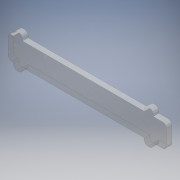
# Autodesk Inventor part: BBGW Case Side
Saved by Autodesk Inventor 2016 (Build 200138000, 138)
## iProperties
Created: 2016-06-26
Part Number: BBGW Case Side
Material: Acrylic, Clear
Document SubType Name: Modeling
Designer: Jacob
Density: 1.19 g/cm^3
Appearance: Transparent - Clear
Author: Jacob
Autodesk Inventor part; units mm, degrees
(part 1 of 2)
ref_plane "YZ Plane" through (0, 0, 0) normal (1, 0, 0) x (0, 1, 0)
ref_plane "XZ Plane" through (0, 0, 0) normal (0, 1, 0) x (-1, 0, 0)
ref_plane "XY Plane" through (0, 0, 0) normal (0, 0, 1) x (1, 0, 0)
sketch "Sketch1" plane through (0, 0, 0) normal (0, 1, 0) x (-1, 0, 0)
  line L0 (176.9998, 77.9421) -> (176.9999, 86.5421)
  spline S0 degree 3 poles (176.9999, 86.5421) (176.9999, 87.6467) (176.1044, 88.5421) (174.9999, 88.5421) knots 0 0 0 0 1 1 1 1
  line L1 (176.9999, 86.5421) -> (176.9999, 87.6467) construction
  line L2 (176.9999, 87.6467) -> (176.1044, 88.5421) construction
  line L3 (176.1044, 88.5421) -> (174.9999, 88.5421) construction
  line L4 (174.9999, 88.5421) -> (173.9998, 88.5421)
  line L5 (173.9998, 88.5421) -> (173.9998, 90.5421)
  line L6 (173.9998, 90.5421) -> (173.9993, 90.5762)
  line L7 (173.9993, 90.5762) -> (173.9975, 90.6103)
  line L8 (173.9975, 90.6103) -> (173.9946, 90.6444)
  line L9 (173.9946, 90.6444) -> (173.9905, 90.6783)
  line L10 (173.9905, 90.6783) -> (173.9853, 90.712)
  line L11 (173.9853, 90.712) -> (173.9789, 90.7456)
  line L12 (173.9789, 90.7456) -> (173.9714, 90.7789)
  line L13 (173.9714, 90.7789) -> (173.9628, 90.8119)
  line L14 (173.9628, 90.8119) -> (173.953, 90.8446)
  line L15 (173.953, 90.8446) -> (173.9421, 90.877)
  line L16 (173.9421, 90.877) -> (173.9301, 90.909)
  line L17 (173.9301, 90.909) -> (173.9171, 90.9405)
  line L18 (173.9171, 90.9405) -> (173.9029, 90.9716)
  line L19 (173.9029, 90.9716) -> (173.8877, 91.0022)
  line L20 (173.8877, 91.0022) -> (173.8715, 91.0322)
  line L21 (173.8715, 91.0322) -> (173.8543, 91.0617)
  line L22 (173.8543, 91.0617) -> (173.836, 91.0906)
  line L23 (173.836, 91.0906) -> (173.8168, 91.1188)
  line L24 (173.8168, 91.1188) -> (173.7967, 91.1463)
  line L25 (173.7967, 91.1463) -> (173.7756, 91.1732)
  line L26 (173.7756, 91.1732) -> (173.7536, 91.1993)
  line L27 (173.7536, 91.1993) -> (173.7307, 91.2247)
  line L28 (173.7307, 91.2247) -> (173.707, 91.2492)
  line L29 (173.707, 91.2492) -> (173.6824, 91.2729)
  line L30 (173.6824, 91.2729) -> (173.6571, 91.2958)
  line L31 (173.6571, 91.2958) -> (173.6309, 91.3178)
  line L32 (173.6309, 91.3178) -> (173.6041, 91.3389)
  line L33 (173.6041, 91.3389) -> (173.5765, 91.3591)
  line L34 (173.5765, 91.3591) -> (173.5483, 91.3783)
  line L35 (173.5483, 91.3783) -> (173.5194, 91.3965)
  line L36 (173.5194, 91.3965) -> (173.49, 91.4138)
  line L37 (173.49, 91.4138) -> (173.4599, 91.43)
  line L38 (173.4599, 91.43) -> (173.4293, 91.4452)
  line L39 (173.4293, 91.4452) -> (173.3983, 91.4593)
  line L40 (173.3983, 91.4593) -> (173.3667, 91.4724)
  line L41 (173.3667, 91.4724) -> (173.3347, 91.4844)
  line L42 (173.3347, 91.4844) -> (173.3024, 91.4952)
  line L43 (173.3024, 91.4952) -> (173.2696, 91.505)
  line L44 (173.2696, 91.505) -> (173.2366, 91.5137)
  line L45 (173.2366, 91.5137) -> (173.2033, 91.5212)
  line L46 (173.2033, 91.5212) -> (173.1698, 91.5276)
  line L47 (173.1698, 91.5276) -> (173.136, 91.5328)
  line L48 (173.136, 91.5328) -> (173.1021, 91.5369)
  line L49 (173.1021, 91.5369) -> (173.0681, 91.5398)
  line L50 (173.0681, 91.5398) -> (173.034, 91.5415)
  line L51 (173.034, 91.5415) -> (172.9999, 91.5421)
  line L52 (172.9999, 91.5421) -> (169.9998, 91.5421)
  line L53 (169.9998, 91.5421) -> (169.9657, 91.5415)
  line L54 (169.9657, 91.5415) -> (169.9316, 91.5398)
  line L55 (169.9316, 91.5398) -> (169.8976, 91.5369)
  line L56 (169.8976, 91.5369) -> (169.8637, 91.5328)
  line L57 (169.8637, 91.5328) -> (169.8299, 91.5276)
  line L58 (169.8299, 91.5276) -> (169.7964, 91.5212)
  line L59 (169.7964, 91.5212) -> (169.7631, 91.5137)
  line L60 (169.7631, 91.5137) -> (169.7301, 91.505)
  line L61 (169.7301, 91.505) -> (169.6973, 91.4952)
  line L62 (169.6973, 91.4952) -> (169.665, 91.4844)
  line L63 (169.665, 91.4844) -> (169.633, 91.4724)
  line L64 (169.633, 91.4724) -> (169.6014, 91.4593)
  line L65 (169.6014, 91.4593) -> (169.5704, 91.4452)
  line L66 (169.5704, 91.4452) -> (169.5398, 91.43)
  line L67 (169.5398, 91.43) -> (169.5097, 91.4138)
  line L68 (169.5097, 91.4138) -> (169.4803, 91.3965)
  line L69 (169.4803, 91.3965) -> (169.4514, 91.3783)
  line L70 (169.4514, 91.3783) -> (169.4232, 91.3591)
  line L71 (169.4232, 91.3591) -> (169.3956, 91.3389)
  line L72 (169.3956, 91.3389) -> (169.3688, 91.3178)
  line L73 (169.3688, 91.3178) -> (169.3426, 91.2958)
  line L74 (169.3426, 91.2958) -> (169.3173, 91.2729)
  line L75 (169.3173, 91.2729) -> (169.2927, 91.2492)
  line L76 (169.2927, 91.2492) -> (169.269, 91.2247)
  line L77 (169.269, 91.2247) -> (169.2461, 91.1993)
  line L78 (169.2461, 91.1993) -> (169.2241, 91.1732)
  line L79 (169.2241, 91.1732) -> (169.203, 91.1463)
  line L80 (169.203, 91.1463) -> (169.1829, 91.1188)
  line L81 (169.1829, 91.1188) -> (169.1637, 91.0906)
  line L82 (169.1637, 91.0906) -> (169.1454, 91.0617)
  line L83 (169.1454, 91.0617) -> (169.1282, 91.0322)
  line L84 (169.1282, 91.0322) -> (169.112, 91.0022)
  line L85 (169.112, 91.0022) -> (169.0968, 90.9716)
  line L86 (169.0968, 90.9716) -> (169.0826, 90.9405)
  line L87 (169.0826, 90.9405) -> (169.0696, 90.909)
  line L88 (169.0696, 90.909) -> (169.0576, 90.877)
  line L89 (169.0576, 90.877) -> (169.0467, 90.8446)
  line L90 (169.0467, 90.8446) -> (169.0369, 90.8119)
  line L91 (169.0369, 90.8119) -> (169.0283, 90.7789)
  line L92 (169.0283, 90.7789) -> (169.0208, 90.7456)
  line L93 (169.0208, 90.7456) -> (169.0144, 90.712)
  line L94 (169.0144, 90.712) -> (169.0092, 90.6783)
  line L95 (169.0092, 90.6783) -> (169.0051, 90.6444)
  line L96 (169.0051, 90.6444) -> (169.0022, 90.6103)
  line L97 (169.0022, 90.6103) -> (169.0004, 90.5762)
  line L98 (169.0004, 90.5762) -> (168.9998, 90.5421)
  line L99 (168.9998, 90.5421) -> (168.9998, 88.5421)
  line L100 (168.9998, 88.5421) -> (102.1834, 88.5421)
  line L101 (102.1834, 88.5421) -> (102.1834, 90.5421)
  line L102 (102.1834, 90.5421) -> (102.1829, 90.5762)
  line L103 (102.1829, 90.5762) -> (102.1811, 90.6103)
  line L104 (102.1811, 90.6103) -> (102.1782, 90.6444)
  line L105 (102.1782, 90.6444) -> (102.1741, 90.6783)
  line L106 (102.1741, 90.6783) -> (102.1689, 90.712)
  line L107 (102.1689, 90.712) -> (102.1625, 90.7456)
  line L108 (102.1625, 90.7456) -> (102.155, 90.7789)
  line L109 (102.155, 90.7789) -> (102.1464, 90.8119)
  line L110 (102.1464, 90.8119) -> (102.1366, 90.8446)
  line L111 (102.1366, 90.8446) -> (102.1257, 90.877)
  line L112 (102.1257, 90.877) -> (102.1137, 90.909)
  line L113 (102.1137, 90.909) -> (102.1007, 90.9405)
  line L114 (102.1007, 90.9405) -> (102.0865, 90.9716)
  line L115 (102.0865, 90.9716) -> (102.0713, 91.0022)
  line L116 (102.0713, 91.0022) -> (102.0551, 91.0322)
  line L117 (102.0551, 91.0322) -> (102.0379, 91.0617)
  line L118 (102.0379, 91.0617) -> (102.0196, 91.0906)
  line L119 (102.0196, 91.0906) -> (102.0004, 91.1188)
  line L120 (102.0004, 91.1188) -> (101.9802, 91.1463)
  line L121 (101.9802, 91.1463) -> (101.9592, 91.1732)
  line L122 (101.9592, 91.1732) -> (101.9372, 91.1993)
  line L123 (101.9372, 91.1993) -> (101.9143, 91.2247)
  line L124 (101.9143, 91.2247) -> (101.8905, 91.2492)
  line L125 (101.8905, 91.2492) -> (101.866, 91.2729)
  line L126 (101.866, 91.2729) -> (101.8406, 91.2958)
  line L127 (101.8406, 91.2958) -> (101.8145, 91.3178)
  line L128 (101.8145, 91.3178) -> (101.7877, 91.3389)
  line L129 (101.7877, 91.3389) -> (101.7601, 91.3591)
  line L130 (101.7601, 91.3591) -> (101.7319, 91.3783)
  line L131 (101.7319, 91.3783) -> (101.703, 91.3965)
  line L132 (101.703, 91.3965) -> (101.6735, 91.4138)
  line L133 (101.6735, 91.4138) -> (101.6435, 91.43)
  line L134 (101.6435, 91.43) -> (101.6129, 91.4452)
  line L135 (101.6129, 91.4452) -> (101.5818, 91.4593)
  line L136 (101.5818, 91.4593) -> (101.5503, 91.4724)
  line L137 (101.5503, 91.4724) -> (101.5183, 91.4844)
  line L138 (101.5183, 91.4844) -> (101.486, 91.4952)
  line L139 (101.486, 91.4952) -> (101.4532, 91.505)
  line L140 (101.4532, 91.505) -> (101.4202, 91.5137)
  line L141 (101.4202, 91.5137) -> (101.3869, 91.5212)
  line L142 (101.3869, 91.5212) -> (101.3533, 91.5276)
  line L143 (101.3533, 91.5276) -> (101.3196, 91.5328)
  line L144 (101.3196, 91.5328) -> (101.2857, 91.5369)
  line L145 (101.2857, 91.5369) -> (101.2517, 91.5398)
  line L146 (101.2517, 91.5398) -> (101.2176, 91.5415)
  line L147 (101.2176, 91.5415) -> (101.1834, 91.5421)
  line L148 (101.1834, 91.5421) -> (98.1834, 91.5421)
  line L149 (98.1834, 91.5421) -> (98.1493, 91.5415)
  line L150 (98.1493, 91.5415) -> (98.1152, 91.5398)
  line L151 (98.1152, 91.5398) -> (98.0812, 91.5369)
  line L152 (98.0812, 91.5369) -> (98.0473, 91.5328)
  line L153 (98.0473, 91.5328) -> (98.0135, 91.5276)
  line L154 (98.0135, 91.5276) -> (97.98, 91.5212)
  line L155 (97.98, 91.5212) -> (97.9467, 91.5137)
  line L156 (97.9467, 91.5137) -> (97.9136, 91.505)
  line L157 (97.9136, 91.505) -> (97.8809, 91.4952)
  line L158 (97.8809, 91.4952) -> (97.8486, 91.4844)
  line L159 (97.8486, 91.4844) -> (97.8166, 91.4724)
  line L160 (97.8166, 91.4724) -> (97.785, 91.4593)
  line L161 (97.785, 91.4593) -> (97.754, 91.4452)
  line L162 (97.754, 91.4452) -> (97.7234, 91.43)
  line L163 (97.7234, 91.43) -> (97.6933, 91.4138)
  line L164 (97.6933, 91.4138) -> (97.6639, 91.3965)
  line L165 (97.6639, 91.3965) -> (97.635, 91.3783)
  line L166 (97.635, 91.3783) -> (97.6068, 91.3591)
  line L167 (97.6068, 91.3591) -> (97.5792, 91.3389)
  line L168 (97.5792, 91.3389) -> (97.5524, 91.3178)
  line L169 (97.5524, 91.3178) -> (97.5262, 91.2958)
  line L170 (97.5262, 91.2958) -> (97.5009, 91.2729)
  line L171 (97.5009, 91.2729) -> (97.4763, 91.2492)
  line L172 (97.4763, 91.2492) -> (97.4526, 91.2247)
  line L173 (97.4526, 91.2247) -> (97.4297, 91.1993)
  line L174 (97.4297, 91.1993) -> (97.4077, 91.1732)
  line L175 (97.4077, 91.1732) -> (97.3866, 91.1463)
  line L176 (97.3866, 91.1463) -> (97.3665, 91.1188)
  line L177 (97.3665, 91.1188) -> (97.3473, 91.0906)
  line L178 (97.3473, 91.0906) -> (97.329, 91.0617)
  line L179 (97.329, 91.0617) -> (97.3118, 91.0322)
  line L180 (97.3118, 91.0322) -> (97.2956, 91.0022)
  line L181 (97.2956, 91.0022) -> (97.2804, 90.9716)
  line L182 (97.2804, 90.9716) -> (97.2662, 90.9405)
  line L183 (97.2662, 90.9405) -> (97.2532, 90.909)
  line L184 (97.2532, 90.909) -> (97.2412, 90.877)
  line L185 (97.2412, 90.877) -> (97.2303, 90.8446)
  line L186 (97.2303, 90.8446) -> (97.2205, 90.8119)
  line L187 (97.2205, 90.8119) -> (97.2119, 90.7789)
  line L188 (97.2119, 90.7789) -> (97.2044, 90.7456)
  line L189 (97.2044, 90.7456) -> (97.198, 90.712)
  line L190 (97.198, 90.712) -> (97.1928, 90.6783)
  line L191 (97.1928, 90.6783) -> (97.1887, 90.6444)
  line L192 (97.1887, 90.6444) -> (97.1858, 90.6103)
  line L193 (97.1858, 90.6103) -> (97.184, 90.5762)
  line L194 (97.184, 90.5762) -> (97.1834, 90.5421)
  line L195 (97.1834, 90.5421) -> (97.1834, 88.5421)
  line L196 (97.1834, 88.5421) -> (92, 88.5421)
  spline S1 degree 3 poles (92, 88.5421) (91.4695, 88.5421) (90.9608, 88.3314) (90.5857, 87.9563) knots 0 0 0 0 0.5 0.5 0.5 0.5
  line L197 (92, 88.5421) -> (91.4695, 88.5421) construction
  line L198 (91.4695, 88.5421) -> (90.9608, 88.3314) construction
  line L199 (90.9608, 88.3314) -> (90.5857, 87.9563) construction
  spline S2 degree 3 poles (90.5857, 87.9563) (90.585325, 87.955925) (90.2107, 87.5812) (90, 87.0725) (90, 86.5421) knots 0.5 0.5 0.5 0.5 0.50000001 1 1 1 1
  line L200 (90.5857, 87.9563) -> (90.5857, 87.9563) construction
  line L201 (90.5857, 87.9563) -> (90.2107, 87.5812) construction
  line L202 (90.2107, 87.5812) -> (90, 87.0725) construction
  line L203 (90, 87.0725) -> (90, 86.5421) construction
  line L204 (90, 86.5421) -> (89.9999, 77.9421)
  spline S3 degree 3 poles (89.9999, 77.9421) (89.9999, 77.4117) (90.2107, 76.903) (90.5857, 76.5279) knots 0 0 0 0 0.5 0.5 0.5 0.5
  line L205 (89.9999, 77.9421) -> (89.9999, 77.4117) construction
  line L206 (89.9999, 77.4117) -> (90.2107, 76.903) construction
  line L207 (90.2107, 76.903) -> (90.5857, 76.5279) construction
  spline S4 degree 3 poles (90.5857, 76.5279) (90.586075, 76.527525) (90.9608, 76.1528) (91.4695, 75.9421) (91.9999, 75.9421) knots 0.5 0.5 0.5 0.5 0.50000001 1 1 1 1
  line L208 (90.5857, 76.5279) -> (90.5857, 76.5279) construction
  line L209 (90.5857, 76.5279) -> (90.9608, 76.1528) construction
  line L210 (90.9608, 76.1528) -> (91.4695, 75.9421) construction
  line L211 (91.4695, 75.9421) -> (91.9999, 75.9421) construction
  line L212 (91.9999, 75.9421) -> (97.1834, 75.9421)
  line L213 (97.1834, 75.9421) -> (97.1834, 73.9421)
  line L214 (97.1834, 73.9421) -> (97.184, 73.908)
  line L215 (97.184, 73.908) -> (97.1858, 73.8739)
  line L216 (97.1858, 73.8739) -> (97.1887, 73.8398)
  line L217 (97.1887, 73.8398) -> (97.1928, 73.8059)
  line L218 (97.1928, 73.8059) -> (97.198, 73.7722)
  line L219 (97.198, 73.7722) -> (97.2044, 73.7386)
  line L220 (97.2044, 73.7386) -> (97.2119, 73.7053)
  line L221 (97.2119, 73.7053) -> (97.2205, 73.6723)
  line L222 (97.2205, 73.6723) -> (97.2303, 73.6396)
  line L223 (97.2303, 73.6396) -> (97.2412, 73.6072)
  line L224 (97.2412, 73.6072) -> (97.2532, 73.5752)
  line L225 (97.2532, 73.5752) -> (97.2662, 73.5437)
  line L226 (97.2662, 73.5437) -> (97.2804, 73.5126)
  line L227 (97.2804, 73.5126) -> (97.2956, 73.482)
  line L228 (97.2956, 73.482) -> (97.3118, 73.452)
  line L229 (97.3118, 73.452) -> (97.329, 73.4225)
  line L230 (97.329, 73.4225) -> (97.3473, 73.3936)
  line L231 (97.3473, 73.3936) -> (97.3665, 73.3654)
  line L232 (97.3665, 73.3654) -> (97.3866, 73.3379)
  line L233 (97.3866, 73.3379) -> (97.4077, 73.311)
  line L234 (97.4077, 73.311) -> (97.4297, 73.2849)
  line L235 (97.4297, 73.2849) -> (97.4526, 73.2595)
  line L236 (97.4526, 73.2595) -> (97.4763, 73.235)
  line L237 (97.4763, 73.235) -> (97.5009, 73.2113)
  line L238 (97.5009, 73.2113) -> (97.5262, 73.1884)
  line L239 (97.5262, 73.1884) -> (97.5524, 73.1664)
  line L240 (97.5524, 73.1664) -> (97.5792, 73.1453)
  line L241 (97.5792, 73.1453) -> (97.6068, 73.1251)
  line L242 (97.6068, 73.1251) -> (97.635, 73.1059)
  line L243 (97.635, 73.1059) -> (97.6639, 73.0877)
  line L244 (97.6639, 73.0877) -> (97.6933, 73.0704)
  line L245 (97.6933, 73.0704) -> (97.7234, 73.0542)
  line L246 (97.7234, 73.0542) -> (97.754, 73.039)
  line L247 (97.754, 73.039) -> (97.785, 73.0249)
  line L248 (97.785, 73.0249) -> (97.8166, 73.0118)
  line L249 (97.8166, 73.0118) -> (97.8486, 72.9998)
  line L250 (97.8486, 72.9998) -> (97.8809, 72.989)
  line L251 (97.8809, 72.989) -> (97.9136, 72.9792)
  line L252 (97.9136, 72.9792) -> (97.9467, 72.9705)
  line L253 (97.9467, 72.9705) -> (97.98, 72.963)
  line L254 (97.98, 72.963) -> (98.0135, 72.9566)
  line L255 (98.0135, 72.9566) -> (98.0473, 72.9514)
  line L256 (98.0473, 72.9514) -> (98.0812, 72.9473)
  line L257 (98.0812, 72.9473) -> (98.1152, 72.9444)
  line L258 (98.1152, 72.9444) -> (98.1493, 72.9427)
  line L259 (98.1493, 72.9427) -> (98.1834, 72.9421)
  line L260 (98.1834, 72.9421) -> (101.1834, 72.9421)
  line L261 (101.1834, 72.9421) -> (101.2176, 72.9427)
  line L262 (101.2176, 72.9427) -> (101.2517, 72.9444)
  line L263 (101.2517, 72.9444) -> (101.2857, 72.9473)
  line L264 (101.2857, 72.9473) -> (101.3196, 72.9514)
  line L265 (101.3196, 72.9514) -> (101.3533, 72.9566)
  line L266 (101.3533, 72.9566) -> (101.3869, 72.963)
  line L267 (101.3869, 72.963) -> (101.4202, 72.9705)
  line L268 (101.4202, 72.9705) -> (101.4532, 72.9792)
  line L269 (101.4532, 72.9792) -> (101.486, 72.989)
  line L270 (101.486, 72.989) -> (101.5183, 72.9998)
  line L271 (101.5183, 72.9998) -> (101.5503, 73.0118)
  line L272 (101.5503, 73.0118) -> (101.5818, 73.0249)
  line L273 (101.5818, 73.0249) -> (101.6129, 73.039)
  line L274 (101.6129, 73.039) -> (101.6435, 73.0542)
  line L275 (101.6435, 73.0542) -> (101.6735, 73.0704)
  line L276 (101.6735, 73.0704) -> (101.703, 73.0877)
  line L277 (101.703, 73.0877) -> (101.7319, 73.1059)
  line L278 (101.7319, 73.1059) -> (101.7601, 73.1251)
  line L279 (101.7601, 73.1251) -> (101.7877, 73.1453)
  line L280 (101.7877, 73.1453) -> (101.8145, 73.1664)
  line L281 (101.8145, 73.1664) -> (101.8406, 73.1884)
  line L282 (101.8406, 73.1884) -> (101.866, 73.2113)
  line L283 (101.866, 73.2113) -> (101.8905, 73.235)
  line L284 (101.8905, 73.235) -> (101.9143, 73.2595)
  line L285 (101.9143, 73.2595) -> (101.9372, 73.2849)
  line L286 (101.9372, 73.2849) -> (101.9592, 73.311)
  line L287 (101.9592, 73.311) -> (101.9802, 73.3379)
  line L288 (101.9802, 73.3379) -> (102.0004, 73.3654)
  line L289 (102.0004, 73.3654) -> (102.0196, 73.3936)
  line L290 (102.0196, 73.3936) -> (102.0379, 73.4225)
  line L291 (102.0379, 73.4225) -> (102.0551, 73.452)
  line L292 (102.0551, 73.452) -> (102.0713, 73.482)
  line L293 (102.0713, 73.482) -> (102.0865, 73.5126)
  line L294 (102.0865, 73.5126) -> (102.1007, 73.5437)
  line L295 (102.1007, 73.5437) -> (102.1137, 73.5752)
  line L296 (102.1137, 73.5752) -> (102.1257, 73.6072)
  line L297 (102.1257, 73.6072) -> (102.1366, 73.6396)
  line L298 (102.1366, 73.6396) -> (102.1464, 73.6723)
  line L299 (102.1464, 73.6723) -> (102.155, 73.7053)
  line L300 (102.155, 73.7053) -> (102.1625, 73.7386)
  line L301 (102.1625, 73.7386) -> (102.1689, 73.7722)
  line L302 (102.1689, 73.7722) -> (102.1741, 73.8059)
  line L303 (102.1741, 73.8059) -> (102.1782, 73.8398)
  line L304 (102.1782, 73.8398) -> (102.1811, 73.8739)
  line L305 (102.1811, 73.8739) -> (102.1829, 73.908)
  line L306 (102.1829, 73.908) -> (102.1834, 73.9421)
  line L307 (102.1834, 73.9421) -> (102.1834, 75.9421)
  line L308 (102.1834, 75.9421) -> (168.9998, 75.9421)
  line L309 (168.9998, 75.9421) -> (168.9998, 73.9421)
  line L310 (168.9998, 73.9421) -> (169.0004, 73.908)
  line L311 (169.0004, 73.908) -> (169.0022, 73.8739)
  line L312 (169.0022, 73.8739) -> (169.0051, 73.8398)
  line L313 (169.0051, 73.8398) -> (169.0092, 73.8059)
  line L314 (169.0092, 73.8059) -> (169.0144, 73.7722)
  line L315 (169.0144, 73.7722) -> (169.0208, 73.7386)
  line L316 (169.0208, 73.7386) -> (169.0283, 73.7053)
  line L317 (169.0283, 73.7053) -> (169.0369, 73.6723)
  line L318 (169.0369, 73.6723) -> (169.0467, 73.6396)
  line L319 (169.0467, 73.6396) -> (169.0576, 73.6072)
  line L320 (169.0576, 73.6072) -> (169.0696, 73.5752)
  line L321 (169.0696, 73.5752) -> (169.0826, 73.5437)
  line L322 (169.0826, 73.5437) -> (169.0968, 73.5126)
  line L323 (169.0968, 73.5126) -> (169.112, 73.482)
  line L324 (169.112, 73.482) -> (169.1282, 73.452)
  line L325 (169.1282, 73.452) -> (169.1454, 73.4225)
  line L326 (169.1454, 73.4225) -> (169.1637, 73.3936)
  line L327 (169.1637, 73.3936) -> (169.1829, 73.3654)
  line L328 (169.1829, 73.3654) -> (169.203, 73.3379)
  line L329 (169.203, 73.3379) -> (169.2241, 73.311)
  line L330 (169.2241, 73.311) -> (169.2461, 73.2849)
  line L331 (169.2461, 73.2849) -> (169.269, 73.2595)
  line L332 (169.269, 73.2595) -> (169.2927, 73.235)
  line L333 (169.2927, 73.235) -> (169.3173, 73.2113)
  line L334 (169.3173, 73.2113) -> (169.3426, 73.1884)
  line L335 (169.3426, 73.1884) -> (169.3688, 73.1664)
  line L336 (169.3688, 73.1664) -> (169.3956, 73.1453)
  line L337 (169.3956, 73.1453) -> (169.4232, 73.1251)
  line L338 (169.4232, 73.1251) -> (169.4514, 73.1059)
  line L339 (169.4514, 73.1059) -> (169.4803, 73.0877)
  line L340 (169.4803, 73.0877) -> (169.5097, 73.0704)
  line L341 (169.5097, 73.0704) -> (169.5398, 73.0542)
  line L342 (169.5398, 73.0542) -> (169.5704, 73.039)
  line L343 (169.5704, 73.039) -> (169.6014, 73.0249)
  line L344 (169.6014, 73.0249) -> (169.633, 73.0118)
  line L345 (169.633, 73.0118) -> (169.665, 72.9998)
  line L346 (169.665, 72.9998) -> (169.6973, 72.989)
  line L347 (169.6973, 72.989) -> (169.7301, 72.9792)
  line L348 (169.7301, 72.9792) -> (169.7631, 72.9705)
  line L349 (169.7631, 72.9705) -> (169.7964, 72.963)
  line L350 (169.7964, 72.963) -> (169.8299, 72.9566)
  line L351 (169.8299, 72.9566) -> (169.8637, 72.9514)
  line L352 (169.8637, 72.9514) -> (169.8976, 72.9473)
  line L353 (169.8976, 72.9473) -> (169.9316, 72.9444)
  line L354 (169.9316, 72.9444) -> (169.9657, 72.9427)
  line L355 (169.9657, 72.9427) -> (169.9998, 72.9421)
  line L356 (169.9998, 72.9421) -> (172.9999, 72.9421)
  line L357 (172.9999, 72.9421) -> (173.034, 72.9427)
  line L358 (173.034, 72.9427) -> (173.0681, 72.9444)
  line L359 (173.0681, 72.9444) -> (173.1021, 72.9473)
  line L360 (173.1021, 72.9473) -> (173.136, 72.9514)
  line L361 (173.136, 72.9514) -> (173.1698, 72.9566)
  line L362 (173.1698, 72.9566) -> (173.2033, 72.963)
  line L363 (173.2033, 72.963) -> (173.2366, 72.9705)
  line L364 (173.2366, 72.9705) -> (173.2696, 72.9792)
  line L365 (173.2696, 72.9792) -> (173.3024, 72.989)
  line L366 (173.3024, 72.989) -> (173.3347, 72.9998)
  line L367 (173.3347, 72.9998) -> (173.3667, 73.0118)
  line L368 (173.3667, 73.0118) -> (173.3983, 73.0249)
  line L369 (173.3983, 73.0249) -> (173.4293, 73.039)
  line L370 (173.4293, 73.039) -> (173.4599, 73.0542)
  line L371 (173.4599, 73.0542) -> (173.49, 73.0704)
  line L372 (173.49, 73.0704) -> (173.5194, 73.0877)
  line L373 (173.5194, 73.0877) -> (173.5483, 73.1059)
  line L374 (173.5483, 73.1059) -> (173.5765, 73.1251)
  line L375 (173.5765, 73.1251) -> (173.6041, 73.1453)
  line L376 (173.6041, 73.1453) -> (173.6309, 73.1664)
  line L377 (173.6309, 73.1664) -> (173.6571, 73.1884)
  line L378 (173.6571, 73.1884) -> (173.6824, 73.2113)
  line L379 (173.6824, 73.2113) -> (173.707, 73.235)
  line L380 (173.707, 73.235) -> (173.7307, 73.2595)
  line L381 (173.7307, 73.2595) -> (173.7536, 73.2849)
  line L382 (173.7536, 73.2849) -> (173.7756, 73.311)
  line L383 (173.7756, 73.311) -> (173.7967, 73.3379)
  line L384 (173.7967, 73.3379) -> (173.8168, 73.3654)
  line L385 (173.8168, 73.3654) -> (173.836, 73.3936)
  line L386 (173.836, 73.3936) -> (173.8543, 73.4225)
  line L387 (173.8543, 73.4225) -> (173.8715, 73.452)
  line L388 (173.8715, 73.452) -> (173.8877, 73.482)
  line L389 (173.8877, 73.482) -> (173.9029, 73.5126)
  line L390 (173.9029, 73.5126) -> (173.9171, 73.5437)
  line L391 (173.9171, 73.5437) -> (173.9301, 73.5752)
  line L392 (173.9301, 73.5752) -> (173.9421, 73.6072)
  line L393 (173.9421, 73.6072) -> (173.953, 73.6396)
  line L394 (173.953, 73.6396) -> (173.9628, 73.6723)
  line L395 (173.9628, 73.6723) -> (173.9714, 73.7053)
  line L396 (173.9714, 73.7053) -> (173.9789, 73.7386)
  line L397 (173.9789, 73.7386) -> (173.9853, 73.7722)
  line L398 (173.9853, 73.7722) -> (173.9905, 73.8059)
  line L399 (173.9905, 73.8059) -> (173.9946, 73.8398)
  line L400 (173.9946, 73.8398) -> (173.9975, 73.8739)
  line L401 (173.9975, 73.8739) -> (173.9993, 73.908)
  line L402 (173.9993, 73.908) -> (173.9999, 73.9421)
  line L403 (173.9999, 73.9421) -> (173.9998, 75.9421)
  line L404 (173.9998, 75.9421) -> (174.9998, 75.9421)
  spline S5 degree 3 poles (174.9999, 75.9421) (176.1044, 75.9421) (176.9998, 76.8375) (176.9998, 77.9421) knots 0 0 0 0 1 1 1 1
  line L405 (174.9999, 75.9421) -> (176.1044, 75.9421) construction
  line L406 (176.1044, 75.9421) -> (176.9998, 76.8375) construction
  line L407 (176.9998, 76.8375) -> (176.9998, 77.9421) construction
  line L408 (87, 77.9421) -> (87.0001, 86.5421)
  spline S6 degree 3 poles (87.0001, 86.5421) (87.0001, 87.6467) (86.1046, 88.5421) (85.0001, 88.5421) knots 0 0 0 0 1 1 1 1
  line L409 (87.0001, 86.5421) -> (87.0001, 87.6467) construction
  line L410 (87.0001, 87.6467) -> (86.1046, 88.5421) construction
  line L411 (86.1046, 88.5421) -> (85.0001, 88.5421) construction
  line L412 (85.0001, 88.5421) -> (84, 88.5421)
  line L413 (84, 88.5415) -> (84, 90.5415)
  line L414 (84, 90.5421) -> (83.9995, 90.5762)
  line L415 (83.9995, 90.5762) -> (83.9977, 90.6103)
  line L416 (83.9977, 90.6103) -> (83.9948, 90.6444)
  line L417 (83.9948, 90.6444) -> (83.9907, 90.6783)
  line L418 (83.9907, 90.6783) -> (83.9855, 90.712)
  line L419 (83.9855, 90.712) -> (83.9791, 90.7456)
  line L420 (83.9791, 90.7456) -> (83.9716, 90.7789)
  line L421 (83.9716, 90.7789) -> (83.963, 90.8119)
  line L422 (83.963, 90.8119) -> (83.9532, 90.8446)
  line L423 (83.9532, 90.8446) -> (83.9423, 90.877)
  line L424 (83.9423, 90.877) -> (83.9303, 90.909)
  line L425 (83.9303, 90.909) -> (83.9173, 90.9405)
  line L426 (83.9173, 90.9405) -> (83.9031, 90.9716)
  line L427 (83.9031, 90.9716) -> (83.8879, 91.0022)
  line L428 (83.8879, 91.0022) -> (83.8717, 91.0322)
  line L429 (83.8717, 91.0322) -> (83.8545, 91.0617)
  line L430 (83.8545, 91.0617) -> (83.8362, 91.0906)
  line L431 (83.8362, 91.0906) -> (83.817, 91.1188)
  line L432 (83.817, 91.1188) -> (83.7969, 91.1463)
  line L433 (83.7969, 91.1463) -> (83.7758, 91.1732)
  line L434 (83.7758, 91.1732) -> (83.7538, 91.1993)
  line L435 (83.7538, 91.1993) -> (83.7309, 91.2247)
  line L436 (83.7309, 91.2247) -> (83.7072, 91.2492)
  line L437 (83.7072, 91.2492) -> (83.6826, 91.2729)
  line L438 (83.6826, 91.2729) -> (83.6573, 91.2958)
  line L439 (83.6573, 91.2958) -> (83.6311, 91.3178)
  line L440 (83.6311, 91.3178) -> (83.6043, 91.3389)
  line L441 (83.6043, 91.3389) -> (83.5767, 91.3591)
  line L442 (83.5767, 91.3591) -> (83.5485, 91.3783)
  line L443 (83.5485, 91.3783) -> (83.5196, 91.3965)
  line L444 (83.5196, 91.3965) -> (83.4902, 91.4138)
  line L445 (83.4902, 91.4138) -> (83.4601, 91.43)
  line L446 (83.4601, 91.43) -> (83.4295, 91.4452)
  line L447 (83.4295, 91.4452) -> (83.3985, 91.4593)
  line L448 (83.3985, 91.4593) -> (83.3669, 91.4724)
  line L449 (83.3669, 91.4724) -> (83.3349, 91.4844)
  line L450 (83.3349, 91.4844) -> (83.3026, 91.4952)
  line L451 (83.3026, 91.4952) -> (83.2698, 91.505)
  line L452 (83.2698, 91.505) -> (83.2368, 91.5137)
  line L453 (83.2368, 91.5137) -> (83.2035, 91.5212)
  line L454 (83.2035, 91.5212) -> (83.17, 91.5276)
  line L455 (83.17, 91.5276) -> (83.1362, 91.5328)
  line L456 (83.1362, 91.5328) -> (83.1023, 91.5369)
  line L457 (83.1023, 91.5369) -> (83.0683, 91.5398)
  line L458 (83.0683, 91.5398) -> (83.0342, 91.5415)
  line L459 (83.0342, 91.5415) -> (83, 91.5421)
  line L460 (83, 91.5421) -> (80, 91.5421)
  line L461 (80, 91.5421) -> (79.9659, 91.5415)
  line L462 (79.9659, 91.5415) -> (79.9318, 91.5398)
  line L463 (79.9318, 91.5398) -> (79.8978, 91.5369)
  line L464 (79.8978, 91.5369) -> (79.8639, 91.5328)
  line L465 (79.8639, 91.5328) -> (79.8301, 91.5276)
  line L466 (79.8301, 91.5276) -> (79.7966, 91.5212)
  line L467 (79.7966, 91.5212) -> (79.7633, 91.5137)
  line L468 (79.7633, 91.5137) -> (79.7303, 91.505)
  line L469 (79.7303, 91.505) -> (79.6975, 91.4952)
  line L470 (79.6975, 91.4952) -> (79.6652, 91.4844)
  line L471 (79.6652, 91.4844) -> (79.6332, 91.4724)
  line L472 (79.6332, 91.4724) -> (79.6016, 91.4593)
  line L473 (79.6016, 91.4593) -> (79.5706, 91.4452)
  line L474 (79.5706, 91.4452) -> (79.54, 91.43)
  line L475 (79.54, 91.43) -> (79.5099, 91.4138)
  line L476 (79.5099, 91.4138) -> (79.4805, 91.3965)
  line L477 (79.4805, 91.3965) -> (79.4516, 91.3783)
  line L478 (79.4516, 91.3783) -> (79.4234, 91.3591)
  line L479 (79.4234, 91.3591) -> (79.3958, 91.3389)
  line L480 (79.3958, 91.3389) -> (79.369, 91.3178)
  line L481 (79.369, 91.3178) -> (79.3428, 91.2958)
  line L482 (79.3428, 91.2958) -> (79.3175, 91.2729)
  line L483 (79.3175, 91.2729) -> (79.2929, 91.2492)
  line L484 (79.2929, 91.2492) -> (79.2692, 91.2247)
  line L485 (79.2692, 91.2247) -> (79.2463, 91.1993)
  line L486 (79.2463, 91.1993) -> (79.2243, 91.1732)
  line L487 (79.2243, 91.1732) -> (79.2032, 91.1463)
  line L488 (79.2032, 91.1463) -> (79.1831, 91.1188)
  line L489 (79.1831, 91.1188) -> (79.1639, 91.0906)
  line L490 (79.1639, 91.0906) -> (79.1456, 91.0617)
  line L491 (79.1456, 91.0617) -> (79.1284, 91.0322)
  line L492 (79.1284, 91.0322) -> (79.1122, 91.0022)
  line L493 (79.1122, 91.0022) -> (79.097, 90.9716)
  line L494 (79.097, 90.9716) -> (79.0828, 90.9405)
  line L495 (79.0828, 90.9405) -> (79.0698, 90.909)
  line L496 (79.0698, 90.909) -> (79.0578, 90.877)
  line L497 (79.0578, 90.877) -> (79.0469, 90.8446)
  line L498 (79.0469, 90.8446) -> (79.0371, 90.8119)
  line L499 (79.0371, 90.8119) -> (79.0285, 90.7789)
  line L500 (79.0285, 90.7789) -> (79.021, 90.7456)
  line L501 (79.021, 90.7456) -> (79.0146, 90.712)
  line L502 (79.0146, 90.712) -> (79.0094, 90.6783)
  line L503 (79.0094, 90.6783) -> (79.0053, 90.6444)
  line L504 (79.0053, 90.6444) -> (79.0024, 90.6103)
  line L505 (79.0024, 90.6103) -> (79.0006, 90.5762)
  line L506 (79.0006, 90.5762) -> (79, 90.5421)
  line L507 (79, 90.5421) -> (79, 88.5421)
  line L508 (79, 88.5421) -> (12.1836, 88.5421)
  line L509 (12.1836, 88.5421) -> (12.1836, 90.5421)
  line L510 (12.1836, 90.5421) -> (12.1831, 90.5762)
  line L511 (12.1831, 90.5762) -> (12.1813, 90.6103)
  line L512 (12.1813, 90.6103) -> (12.1784, 90.6444)
  line L513 (12.1784, 90.6444) -> (12.1743, 90.6783)
  line L514 (12.1743, 90.6783) -> (12.1691, 90.712)
  line L515 (12.1691, 90.712) -> (12.1627, 90.7456)
  line L516 (12.1627, 90.7456) -> (12.1552, 90.7789)
  line L517 (12.1552, 90.7789) -> (12.1466, 90.8119)
  line L518 (12.1466, 90.8119) -> (12.1368, 90.8446)
  line L519 (12.1368, 90.8446) -> (12.1259, 90.877)
  line L520 (12.1259, 90.877) -> (12.1139, 90.909)
  line L521 (12.1139, 90.909) -> (12.1009, 90.9405)
  line L522 (12.1009, 90.9405) -> (12.0867, 90.9716)
  line L523 (12.0867, 90.9716) -> (12.0715, 91.0022)
  line L524 (12.0715, 91.0022) -> (12.0553, 91.0322)
  line L525 (12.0553, 91.0322) -> (12.0381, 91.0617)
  line L526 (12.0381, 91.0617) -> (12.0198, 91.0906)
  line L527 (12.0198, 91.0906) -> (12.0006, 91.1188)
  line L528 (12.0006, 91.1188) -> (11.9804, 91.1463)
  line L529 (11.9804, 91.1463) -> (11.9594, 91.1732)
  line L530 (11.9594, 91.1732) -> (11.9374, 91.1993)
  line L531 (11.9374, 91.1993) -> (11.9145, 91.2247)
  line L532 (11.9145, 91.2247) -> (11.8907, 91.2492)
  line L533 (11.8907, 91.2492) -> (11.8662, 91.2729)
  line L534 (11.8662, 91.2729) -> (11.8408, 91.2958)
  line L535 (11.8408, 91.2958) -> (11.8147, 91.3178)
  line L536 (11.8147, 91.3178) -> (11.7879, 91.3389)
  line L537 (11.7879, 91.3389) -> (11.7603, 91.3591)
  line L538 (11.7603, 91.3591) -> (11.7321, 91.3783)
  line L539 (11.7321, 91.3783) -> (11.7032, 91.3965)
  line L540 (11.7032, 91.3965) -> (11.6737, 91.4138)
  line L541 (11.6737, 91.4138) -> (11.6437, 91.43)
  line L542 (11.6437, 91.43) -> (11.6131, 91.4452)
  line L543 (11.6131, 91.4452) -> (11.582, 91.4593)
  line L544 (11.582, 91.4593) -> (11.5505, 91.4724)
  line L545 (11.5505, 91.4724) -> (11.5185, 91.4844)
  line L546 (11.5185, 91.4844) -> (11.4862, 91.4952)
  line L547 (11.4862, 91.4952) -> (11.4534, 91.505)
  line L548 (11.4534, 91.505) -> (11.4204, 91.5137)
  line L549 (11.4204, 91.5137) -> (11.3871, 91.5212)
  line L550 (11.3871, 91.5212) -> (11.3535, 91.5276)
  line L551 (11.3535, 91.5276) -> (11.3198, 91.5328)
  line L552 (11.3198, 91.5328) -> (11.2859, 91.5369)
  line L553 (11.2859, 91.5369) -> (11.2519, 91.5398)
  line L554 (11.2519, 91.5398) -> (11.2178, 91.5415)
  line L555 (11.2178, 91.5415) -> (11.1836, 91.5421)
  line L556 (11.1836, 91.5421) -> (8.1836, 91.5421)
  line L557 (8.1836, 91.5421) -> (8.1495, 91.5415)
  line L558 (8.1495, 91.5415) -> (8.1154, 91.5398)
  line L559 (8.1154, 91.5398) -> (8.0814, 91.5369)
  line L560 (8.0814, 91.5369) -> (8.0475, 91.5328)
  line L561 (8.0475, 91.5328) -> (8.0137, 91.5276)
  line L562 (8.0137, 91.5276) -> (7.9802, 91.5212)
  line L563 (7.9802, 91.5212) -> (7.9469, 91.5137)
  line L564 (7.9469, 91.5137) -> (7.9138, 91.505)
  line L565 (7.9138, 91.505) -> (7.8811, 91.4952)
  line L566 (7.8811, 91.4952) -> (7.8488, 91.4844)
  line L567 (7.8488, 91.4844) -> (7.8168, 91.4724)
  line L568 (7.8168, 91.4724) -> (7.7852, 91.4593)
  line L569 (7.7852, 91.4593) -> (7.7542, 91.4452)
  line L570 (7.7542, 91.4452) -> (7.7236, 91.43)
  line L571 (7.7236, 91.43) -> (7.6935, 91.4138)
  line L572 (7.6935, 91.4138) -> (7.6641, 91.3965)
  line L573 (7.6641, 91.3965) -> (7.6352, 91.3783)
  line L574 (7.6352, 91.3783) -> (7.607, 91.3591)
  line L575 (7.607, 91.3591) -> (7.5794, 91.3389)
  line L576 (7.5794, 91.3389) -> (7.5526, 91.3178)
  line L577 (7.5526, 91.3178) -> (7.5264, 91.2958)
  line L578 (7.5264, 91.2958) -> (7.5011, 91.2729)
  line L579 (7.5011, 91.2729) -> (7.4765, 91.2492)
  line L580 (7.4765, 91.2492) -> (7.4528, 91.2247)
  line L581 (7.4528, 91.2247) -> (7.4299, 91.1993)
  line L582 (7.4299, 91.1993) -> (7.4079, 91.1732)
  line L583 (7.4079, 91.1732) -> (7.3868, 91.1463)
  line L584 (7.3868, 91.1463) -> (7.3667, 91.1188)
  line L585 (7.3667, 91.1188) -> (7.3475, 91.0906)
  line L586 (7.3475, 91.0906) -> (7.3292, 91.0617)
  line L587 (7.3292, 91.0617) -> (7.312, 91.0322)
  line L588 (7.312, 91.0322) -> (7.2958, 91.0022)
  line L589 (7.2958, 91.0022) -> (7.2806, 90.9716)
  line L590 (7.2806, 90.9716) -> (7.2664, 90.9405)
  line L591 (7.2664, 90.9405) -> (7.2534, 90.909)
  line L592 (7.2534, 90.909) -> (7.2414, 90.877)
  line L593 (7.2414, 90.877) -> (7.2305, 90.8446)
  line L594 (7.2305, 90.8446) -> (7.2207, 90.8119)
  line L595 (7.2207, 90.8119) -> (7.2121, 90.7789)
  line L596 (7.2121, 90.7789) -> (7.2046, 90.7456)
  line L597 (7.2046, 90.7456) -> (7.1982, 90.712)
  line L598 (7.1982, 90.712) -> (7.193, 90.6783)
  line L599 (7.193, 90.6783) -> (7.1889, 90.6444)
  line L600 (7.1889, 90.6444) -> (7.186, 90.6103)
  line L601 (7.186, 90.6103) -> (7.1842, 90.5762)
  line L602 (7.1842, 90.5762) -> (7.1836, 90.5421)
  line L603 (7.1836, 90.5421) -> (7.1836, 88.5421)
  line L604 (7.1836, 88.5421) -> (2.0001, 88.5421)
  spline S7 degree 3 poles (2.0001, 88.5421) (1.4696, 88.5421) (0.9609, 88.3314) (0.5858, 87.9563) knots 0 0 0 0 0.5 0.5 0.5 0.5
  line L605 (2.0001, 88.5421) -> (1.4696, 88.5421) construction
  line L606 (1.4696, 88.5421) -> (0.9609, 88.3314) construction
  line L607 (0.9609, 88.3314) -> (0.5858, 87.9563) construction
  spline S8 degree 3 poles (0.5858, 87.9563) (0.585425, 87.955925) (0.2108, 87.5812) (0.0001, 87.0725) (0.0001, 86.5421) knots 0.5 0.5 0.5 0.5 0.50000001 1 1 1 1
  line L608 (0.5858, 87.9563) -> (0.5858, 87.9563) construction
  line L609 (0.5858, 87.9563) -> (0.2108, 87.5812) construction
  line L610 (0.2108, 87.5812) -> (0.0001, 87.0725) construction
  line L611 (0.0001, 87.0725) -> (0.0001, 86.5421) construction
  line L612 (0.0001, 86.5421) -> (0, 77.9421)
  spline S9 degree 3 poles (-0.00044, 77.9421) (-0.000303, 77.4117) (0.21063, 76.903055) (0.585727, 76.528052) knots 0 0 0 0 0.5 0.5 0.5 0.5
  line L613 (-0.00044, 77.9421) -> (-0.000303, 77.4117) construction
  line L614 (-0.000303, 77.4117) -> (0.21063, 76.903055) construction
  line L615 (0.21063, 76.903055) -> (0.585727, 76.528052) construction
  spline S10 degree 3 poles (0.5858, 76.5279) (0.586175, 76.527525) (0.9609, 76.1528) (1.4696, 75.9421) (2, 75.9421) knots 0.5 0.5 0.5 0.5 0.50000001 1 1 1 1
  line L616 (0.5858, 76.5279) -> (0.5858, 76.5279) construction
  line L617 (0.5858, 76.5279) -> (0.9609, 76.1528) construction
  line L618 (0.9609, 76.1528) -> (1.4696, 75.9421) construction
  line L619 (1.4696, 75.9421) -> (2, 75.9421) construction
  line L620 (2, 75.9421) -> (7.1836, 75.9421)
  line L621 (7.18414, 75.9421) -> (7.18414, 73.9421)
  line L622 (7.1836, 73.9421) -> (7.1842, 73.908)
  line L623 (7.1842, 73.908) -> (7.186, 73.8739)
  line L624 (7.186, 73.8739) -> (7.1889, 73.8398)
  line L625 (7.1889, 73.8398) -> (7.193, 73.8059)
  line L626 (7.193, 73.8059) -> (7.1982, 73.7722)
  line L627 (7.1982, 73.7722) -> (7.2046, 73.7386)
  line L628 (7.2046, 73.7386) -> (7.2121, 73.7053)
  line L629 (7.2121, 73.7053) -> (7.2207, 73.6723)
  line L630 (7.2207, 73.6723) -> (7.2305, 73.6396)
  line L631 (7.2305, 73.6396) -> (7.2414, 73.6072)
  line L632 (7.2414, 73.6072) -> (7.2534, 73.5752)
  line L633 (7.2534, 73.5752) -> (7.2664, 73.5437)
  line L634 (7.2664, 73.5437) -> (7.2806, 73.5126)
  line L635 (7.2806, 73.5126) -> (7.2958, 73.482)
  line L636 (7.2958, 73.482) -> (7.312, 73.452)
  line L637 (7.312, 73.452) -> (7.3292, 73.4225)
  line L638 (7.3292, 73.4225) -> (7.3475, 73.3936)
  line L639 (7.3475, 73.3936) -> (7.3667, 73.3654)
  line L640 (7.3667, 73.3654) -> (7.3868, 73.3379)
  line L641 (7.3868, 73.3379) -> (7.4079, 73.311)
  line L642 (7.4079, 73.311) -> (7.4299, 73.2849)
  line L643 (7.4299, 73.2849) -> (7.4528, 73.2595)
  line L644 (7.4528, 73.2595) -> (7.4765, 73.235)
  line L645 (7.4765, 73.235) -> (7.5011, 73.2113)
  line L646 (7.5011, 73.2113) -> (7.5264, 73.1884)
  line L647 (7.5264, 73.1884) -> (7.5526, 73.1664)
  line L648 (7.5526, 73.1664) -> (7.5794, 73.1453)
  line L649 (7.5794, 73.1453) -> (7.607, 73.1251)
  line L650 (7.607, 73.1251) -> (7.6352, 73.1059)
  line L651 (7.6352, 73.1059) -> (7.6641, 73.0877)
  line L652 (7.6641, 73.0877) -> (7.6935, 73.0704)
  line L653 (7.6935, 73.0704) -> (7.7236, 73.0542)
  line L654 (7.7236, 73.0542) -> (7.7542, 73.039)
  line L655 (7.7542, 73.039) -> (7.7852, 73.0249)
  line L656 (7.7852, 73.0249) -> (7.8168, 73.0118)
  line L657 (7.8168, 73.0118) -> (7.8488, 72.9998)
  line L658 (7.8488, 72.9998) -> (7.8811, 72.989)
  line L659 (7.8811, 72.989) -> (7.9138, 72.9792)
  line L660 (7.9138, 72.9792) -> (7.9469, 72.9705)
  line L661 (7.9469, 72.9705) -> (7.9802, 72.963)
  line L662 (7.9802, 72.963) -> (8.0137, 72.9566)
  line L663 (8.0137, 72.9566) -> (8.0475, 72.9514)
  line L664 (8.0475, 72.9514) -> (8.0814, 72.9473)
  line L665 (8.0814, 72.9473) -> (8.1154, 72.9444)
  line L666 (8.1154, 72.9444) -> (8.1495, 72.9427)
  line L667 (8.1495, 72.9427) -> (8.1836, 72.9421)
  line L668 (8.1836, 72.9421) -> (11.1836, 72.9421)
  line L669 (11.18414, 72.9421) -> (11.21834, 72.9427)
  line L670 (11.2178, 72.9427) -> (11.2519, 72.9444)
  line L671 (11.2519, 72.9444) -> (11.2859, 72.9473)
  line L672 (11.2859, 72.9473) -> (11.3198, 72.9514)
  line L673 (11.3198, 72.9514) -> (11.3535, 72.9566)
  line L674 (11.3535, 72.9566) -> (11.3871, 72.963)
  line L675 (11.3871, 72.963) -> (11.4204, 72.9705)
  line L676 (11.4204, 72.9705) -> (11.4534, 72.9792)
  line L677 (11.4534, 72.9792) -> (11.4862, 72.989)
  line L678 (11.4862, 72.989) -> (11.5185, 72.9998)
  line L679 (11.5185, 72.9998) -> (11.5505, 73.0118)
  line L680 (11.5505, 73.0118) -> (11.582, 73.0249)
  line L681 (11.582, 73.0249) -> (11.6131, 73.039)
  line L682 (11.6131, 73.039) -> (11.6437, 73.0542)
  line L683 (11.6437, 73.0542) -> (11.6737, 73.0704)
  line L684 (11.6737, 73.0704) -> (11.7032, 73.0877)
  line L685 (11.7032, 73.0877) -> (11.7321, 73.1059)
  line L686 (11.7321, 73.1059) -> (11.7603, 73.1251)
  line L687 (11.7603, 73.1251) -> (11.7879, 73.1453)
  line L688 (11.7879, 73.1453) -> (11.8147, 73.1664)
  line L689 (11.8147, 73.1664) -> (11.8408, 73.1884)
  line L690 (11.8408, 73.1884) -> (11.8662, 73.2113)
  line L691 (11.8662, 73.2113) -> (11.8907, 73.235)
  line L692 (11.8907, 73.235) -> (11.9145, 73.2595)
  line L693 (11.9145, 73.2595) -> (11.9374, 73.2849)
  line L694 (11.9374, 73.2849) -> (11.9594, 73.311)
  line L695 (11.9594, 73.311) -> (11.9804, 73.3379)
  line L696 (11.9804, 73.3379) -> (12.0006, 73.3654)
  line L697 (12.0006, 73.3654) -> (12.0198, 73.3936)
  line L698 (12.0198, 73.3936) -> (12.0381, 73.4225)
  line L699 (12.0381, 73.4225) -> (12.0553, 73.452)
  line L700 (12.0553, 73.452) -> (12.0715, 73.482)
  line L701 (12.0715, 73.482) -> (12.0867, 73.5126)
  line L702 (12.0867, 73.5126) -> (12.1009, 73.5437)
  line L703 (12.1009, 73.5437) -> (12.1139, 73.5752)
  line L704 (12.1139, 73.5752) -> (12.1259, 73.6072)
  line L705 (12.1259, 73.6072) -> (12.1368, 73.6396)
  line L706 (12.1368, 73.6396) -> (12.1466, 73.6723)
  line L707 (12.1466, 73.6723) -> (12.1552, 73.7053)
  line L708 (12.1552, 73.7053) -> (12.1627, 73.7386)
  line L709 (12.1627, 73.7386) -> (12.1691, 73.7722)
  line L710 (12.1691, 73.7722) -> (12.1743, 73.8059)
  line L711 (12.1743, 73.8059) -> (12.1784, 73.8398)
  line L712 (12.1784, 73.8398) -> (12.1813, 73.8739)
  line L713 (12.1813, 73.8739) -> (12.1831, 73.908)
  line L714 (12.1831, 73.908) -> (12.1836, 73.9421)
  line L715 (12.1836, 73.9421) -> (12.1836, 75.9421)
  line L716 (12.18414, 75.9421) -> (79.00054, 75.9421)
  line L717 (79.00054, 75.9421) -> (79.00054, 73.9421)
  line L718 (79, 73.9421) -> (79.0006, 73.908)
  line L719 (79.0006, 73.908) -> (79.0024, 73.8739)
  line L720 (79.0024, 73.8739) -> (79.0053, 73.8398)
  line L721 (79.0053, 73.8398) -> (79.0094, 73.8059)
  line L722 (79.0094, 73.8059) -> (79.0146, 73.7722)
  line L723 (79.0146, 73.7722) -> (79.021, 73.7386)
  line L724 (79.021, 73.7386) -> (79.0285, 73.7053)
  line L725 (79.0285, 73.7053) -> (79.0371, 73.6723)
  line L726 (79.0371, 73.6723) -> (79.0469, 73.6396)
  line L727 (79.0469, 73.6396) -> (79.0578, 73.6072)
  line L728 (79.0578, 73.6072) -> (79.0698, 73.5752)
  line L729 (79.0698, 73.5752) -> (79.0828, 73.5437)
  line L730 (79.0828, 73.5437) -> (79.097, 73.5126)
  line L731 (79.097, 73.5126) -> (79.1122, 73.482)
  line L732 (79.1122, 73.482) -> (79.1284, 73.452)
  line L733 (79.1284, 73.452) -> (79.1456, 73.4225)
  line L734 (79.1456, 73.4225) -> (79.1639, 73.3936)
  line L735 (79.1639, 73.3936) -> (79.1831, 73.3654)
  line L736 (79.1831, 73.3654) -> (79.2032, 73.3379)
  line L737 (79.2032, 73.3379) -> (79.2243, 73.311)
  line L738 (79.2243, 73.311) -> (79.2463, 73.2849)
  line L739 (79.2463, 73.2849) -> (79.2692, 73.2595)
  line L740 (79.2692, 73.2595) -> (79.2929, 73.235)
  line L741 (79.2929, 73.235) -> (79.3175, 73.2113)
  line L742 (79.3175, 73.2113) -> (79.3428, 73.1884)
  line L743 (79.3428, 73.1884) -> (79.369, 73.1664)
  line L744 (79.369, 73.1664) -> (79.3958, 73.1453)
  line L745 (79.3958, 73.1453) -> (79.4234, 73.1251)
  line L746 (79.4234, 73.1251) -> (79.4516, 73.1059)
  line L747 (79.4516, 73.1059) -> (79.4805, 73.0877)
  line L748 (79.4805, 73.0877) -> (79.5099, 73.0704)
  line L749 (79.5099, 73.0704) -> (79.54, 73.0542)
  line L750 (79.54, 73.0542) -> (79.5706, 73.039)
  line L751 (79.5706, 73.039) -> (79.6016, 73.0249)
  line L752 (79.6016, 73.0249) -> (79.6332, 73.0118)
  line L753 (79.6332, 73.0118) -> (79.6652, 72.9998)
  line L754 (79.6652, 72.9998) -> (79.6975, 72.989)
  line L755 (79.6975, 72.989) -> (79.7303, 72.9792)
  line L756 (79.7303, 72.9792) -> (79.7633, 72.9705)
  line L757 (79.7633, 72.9705) -> (79.7966, 72.963)
  line L758 (79.7966, 72.963) -> (79.8301, 72.9566)
  line L759 (79.8301, 72.9566) -> (79.8639, 72.9514)
  line L760 (79.8639, 72.9514) -> (79.8978, 72.9473)
  line L761 (79.8978, 72.9473) -> (79.9318, 72.9444)
  line L762 (79.9318, 72.9444) -> (79.9659, 72.9427)
  line L763 (79.9659, 72.9427) -> (80, 72.9421)
  line L764 (80, 72.9421) -> (83.0001, 72.9421)
  line L765 (83.0002, 72.9421) -> (83.0343, 72.9427)
  line L766 (83.0342, 72.9427) -> (83.0683, 72.9444)
  line L767 (83.0683, 72.9444) -> (83.1023, 72.9473)
  line L768 (83.1023, 72.9473) -> (83.1362, 72.9514)
  line L769 (83.1362, 72.9514) -> (83.17, 72.9566)
  line L770 (83.17, 72.9566) -> (83.2035, 72.963)
  line L771 (83.2035, 72.963) -> (83.2368, 72.9705)
  line L772 (83.2368, 72.9705) -> (83.2698, 72.9792)
  line L773 (83.2698, 72.9792) -> (83.3026, 72.989)
  line L774 (83.3026, 72.989) -> (83.3349, 72.9998)
  line L775 (83.3349, 72.9998) -> (83.3669, 73.0118)
  line L776 (83.3669, 73.0118) -> (83.3985, 73.0249)
  line L777 (83.3985, 73.0249) -> (83.4295, 73.039)
  line L778 (83.4295, 73.039) -> (83.4601, 73.0542)
  line L779 (83.4601, 73.0542) -> (83.4902, 73.0704)
  line L780 (83.4902, 73.0704) -> (83.5196, 73.0877)
  line L781 (83.5196, 73.0877) -> (83.5485, 73.1059)
  line L782 (83.5485, 73.1059) -> (83.5767, 73.1251)
  line L783 (83.5767, 73.1251) -> (83.6043, 73.1453)
  line L784 (83.6043, 73.1453) -> (83.6311, 73.1664)
  line L785 (83.6311, 73.1664) -> (83.6573, 73.1884)
  line L786 (83.6573, 73.1884) -> (83.6826, 73.2113)
  line L787 (83.6826, 73.2113) -> (83.7072, 73.235)
  line L788 (83.7072, 73.235) -> (83.7309, 73.2595)
  line L789 (83.7309, 73.2595) -> (83.7538, 73.2849)
  line L790 (83.7538, 73.2849) -> (83.7758, 73.311)
  line L791 (83.7758, 73.311) -> (83.7969, 73.3379)
  line L792 (83.7969, 73.3379) -> (83.817, 73.3654)
  line L793 (83.817, 73.3654) -> (83.8362, 73.3936)
  line L794 (83.8362, 73.3936) -> (83.8545, 73.4225)
  line L795 (83.8545, 73.4225) -> (83.8717, 73.452)
  line L796 (83.8717, 73.452) -> (83.8879, 73.482)
  line L797 (83.8879, 73.482) -> (83.9031, 73.5126)
  line L798 (83.9031, 73.5126) -> (83.9173, 73.5437)
  line L799 (83.9173, 73.5437) -> (83.9303, 73.5752)
  line L800 (83.9303, 73.5752) -> (83.9423, 73.6072)
  line L801 (83.9423, 73.6072) -> (83.9532, 73.6396)
  line L802 (83.9532, 73.6396) -> (83.963, 73.6723)
  line L803 (83.963, 73.6723) -> (83.9716, 73.7053)
  line L804 (83.9716, 73.7053) -> (83.9791, 73.7386)
  line L805 (83.9791, 73.7386) -> (83.9855, 73.7722)
  line L806 (83.9855, 73.7722) -> (83.9907, 73.8059)
  line L807 (83.9907, 73.8059) -> (83.9948, 73.8398)
  line L808 (83.9948, 73.8398) -> (83.9977, 73.8739)
  line L809 (83.9977, 73.8739) -> (83.9995, 73.908)
  line L810 (83.9995, 73.908) -> (84.0001, 73.9421)
  line L811 (84.0001, 73.9421) -> (84, 75.9421)
  line L812 (84.0001, 75.9421) -> (85.0001, 75.9421)
  spline S11 degree 3 poles (85, 75.9421) (86.1046, 75.9421) (87, 76.8375) (87, 77.9421) knots 0 0 0 0 1 1 1 1
  line L813 (85, 75.9421) -> (86.1046, 75.9421) construction
  line L814 (86.1046, 75.9421) -> (87, 76.8375) construction
  line L815 (87, 76.8375) -> (87, 77.9421) construction
  line L816 (9, 22.3081) -> (7, 22.3081)
  line L817 (7, 22.0081) -> (9, 22.0081)
  line L818 (7, 22.3081) -> (7, 24.3081)
  line L819 (7, 24.3081) -> (6, 24.3081)
  line L820 (6, 24.3081) -> (6, 28.3081)
  spline S12 degree 3 poles (6, 28.3081) (6, 28.5734) (5.8947, 28.8277) (5.7072, 29.0153) knots 0 0 0 0 0.5 0.5 0.5 0.5
  line L821 (6, 28.3081) -> (6, 28.5734) construction
  line L822 (6, 28.5734) -> (5.8947, 28.8277) construction
  line L823 (5.8947, 28.8277) -> (5.7072, 29.0153) construction
  spline S13 degree 3 poles (5.7072, 29.0153) (5.707012, 29.015488) (5.5196, 29.2028) (5.2653, 29.3081) (5, 29.3081) knots 0.5 0.5 0.5 0.5 0.50000001 1 1 1 1
  line L824 (5.7072, 29.0153) -> (5.7072, 29.0153) construction
  line L825 (5.7072, 29.0153) -> (5.5196, 29.2028) construction
  line L826 (5.5196, 29.2028) -> (5.2653, 29.3081) construction
  line L827 (5.2653, 29.3081) -> (5, 29.3081) construction
  line L828 (5, 29.3081) -> (3, 29.3081)
  spline S14 degree 3 poles (3, 29.3081) (2.7348, 29.3081) (2.4805, 29.2028) (2.2929, 29.0153) knots 0 0 0 0 0.5 0.5 0.5 0.5
  line L829 (3, 29.3081) -> (2.7348, 29.3081) construction
  line L830 (2.7348, 29.3081) -> (2.4805, 29.2028) construction
  line L831 (2.4805, 29.2028) -> (2.2929, 29.0153) construction
  spline S15 degree 3 poles (2.2929, 29.0153) (2.292713, 29.015112) (2.1054, 28.8277) (2, 28.5734) (2, 28.3081) knots 0.5 0.5 0.5 0.5 0.50000001 1 1 1 1
  line L832 (2.2929, 29.0153) -> (2.2929, 29.0153) construction
  line L833 (2.2929, 29.0153) -> (2.1054, 28.8277) construction
  line L834 (2.1054, 28.8277) -> (2, 28.5734) construction
  line L835 (2, 28.5734) -> (2, 28.3081) construction
  line L836 (2, 28.3081) -> (2, 24.3081)
  line L837 (2, 24.3081) -> (1, 24.3081)
  line L838 (1, 24.3081) -> (1, 20.6081)
  line L839 (1, 20.6081) -> (7, 20.6081)
  line L840 (7, 20.6081) -> (7, 22.0081)
  line L841 (9, 22.0081) -> (9, 20.6081)
  line L842 (9, 20.6081) -> (15, 20.6081)
  line L843 (15, 20.6081) -> (15, 24.3081)
  line L844 (15, 24.3081) -> (14, 24.3081)
  line L845 (14, 24.3081) -> (14, 28.3081)
  spline S16 degree 3 poles (14, 28.3081) (14, 28.5734) (13.8947, 28.8277) (13.7072, 29.0153) knots 0 0 0 0 0.5 0.5 0.5 0.5
  line L846 (14, 28.3081) -> (14, 28.5734) construction
  line L847 (14, 28.5734) -> (13.8947, 28.8277) construction
  line L848 (13.8947, 28.8277) -> (13.7072, 29.0153) construction
  spline S17 degree 3 poles (13.7072, 29.0153) (13.707012, 29.015488) (13.5196, 29.2028) (13.2653, 29.3081) (13, 29.3081) knots 0.5 0.5 0.5 0.5 0.50000001 1 1 1 1
  line L849 (13.7072, 29.0153) -> (13.7072, 29.0153) construction
  line L850 (13.7072, 29.0153) -> (13.5196, 29.2028) construction
  line L851 (13.5196, 29.2028) -> (13.2653, 29.3081) construction
  line L852 (13.2653, 29.3081) -> (13, 29.3081) construction
  line L853 (13, 29.3081) -> (11, 29.3081)
  spline S18 degree 3 poles (11, 29.3081) (10.7348, 29.3081) (10.4805, 29.2028) (10.2929, 29.0153) knots 0 0 0 0 0.5 0.5 0.5 0.5
  line L854 (11, 29.3081) -> (10.7348, 29.3081) construction
  line L855 (10.7348, 29.3081) -> (10.4805, 29.2028) construction
  line L856 (10.4805, 29.2028) -> (10.2929, 29.0153) construction
  spline S19 degree 3 poles (10.2929, 29.0153) (10.292713, 29.015112) (10.1054, 28.8277) (10, 28.5734) (10, 28.3081) knots 0.5 0.5 0.5 0.5 0.50000001 1 1 1 1
  line L857 (10.2929, 29.0153) -> (10.2929, 29.0153) construction
  line L858 (10.2929, 29.0153) -> (10.1054, 28.8277) construction
  line L859 (10.1054, 28.8277) -> (10, 28.5734) construction
  line L860 (10, 28.5734) -> (10, 28.3081) construction
  line L861 (10, 28.3081) -> (10, 24.3081)
  line L862 (10, 24.3081) -> (9, 24.3081)
  line L863 (9, 24.3081) -> (9, 22.3081)
  line L864 (9, 39.0081) -> (9, 37.6081)
  line L865 (9, 37.6081) -> (15, 37.6081)
  line L866 (15, 37.6081) -> (15, 41.3081)
  line L867 (15, 41.3081) -> (14, 41.3081)
  line L868 (14, 41.3081) -> (14, 45.308)
  spline S20 degree 3 poles (14, 45.308) (14, 45.5733) (13.8947, 45.8276) (13.7072, 46.0152) knots 0 0 0 0 0.5 0.5 0.5 0.5
  line L869 (14, 45.308) -> (14, 45.5733) construction